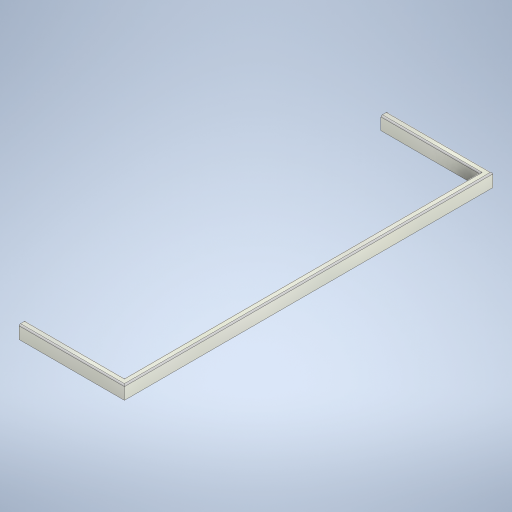
# Autodesk Inventor part: 矮牆
Saved by Autodesk Inventor 2024.2 (Build 282272000, 272)
## iProperties
Created: 2024-06-05
Part Number: 矮牆
Material: 一般
Document SubType Name: Modeling
Designer: User
Density: 1 g/cm^3
Appearance: 預設
Author: User
Autodesk Inventor part; units mm, degrees
ref_plane "YZ Plane" through (0, 0, 0) normal (1, 0, 0) x (0, 1, 0)
ref_plane "XZ Plane" through (0, 0, 0) normal (0, 1, 0) x (-1, 0, 0)
ref_plane "XY Plane" through (0, 0, 0) normal (0, 0, 1) x (1, 0, 0)
sketch "草圖1" plane through (0, 0, 0) normal (0, 1, 0) x (-1, 0, 0)
  line L0 (-8, 28) -> (-8, -28)
  line L1 (-8, -28) -> (8, -28)
  line L2 (8, -28) -> (8, 28)
  line L3 (8, 28) -> (-8, 28)
  line L4 (-8, 28) -> (8, -28) construction
  line L5 (-8, -28) -> (8, 28) construction
  line L6 (-7, 27) -> (-7, -27)
  line L7 (-7, -27) -> (7, -27)
  line L8 (7, -27) -> (7, 27)
  line L9 (7, 27) -> (-7, 27)
  line L10 (-7, 27) -> (7, -27) construction
  line L11 (-7, -27) -> (7, 27) construction
  line L12 (7, 27) -> (8, 27)
  line L13 (7, -27) -> (8, -27)
  point P0 (0, 0)
  dimension "d0" = 56
  dimension "d1" = 16
  dimension "d2" = 54
  dimension "d3" = 14
  constraints: 28 end point, 5 parallel, 4 midpoint, 4 perpendicular, 2 point on line, 1 vertical
  measures "d0" distance of L0.start L0.end
  measures "d1" distance of L1.end L0.end
  measures "d2" distance of L6.start L6.end
  measures "d3" distance of L7.end L6.end
extrude "擠出1" add sketch "草圖1" along normal blind 2 contours L3 L2 L12 L9 L6 L7 L13 L1 L0
fillet "圓角1" radius 0.2 6 edges at (0, 2, 27) (7, 2, 0) (8, 2, 0) (0, 2, 28) (0, 2, -27) (0, 2, -28)
